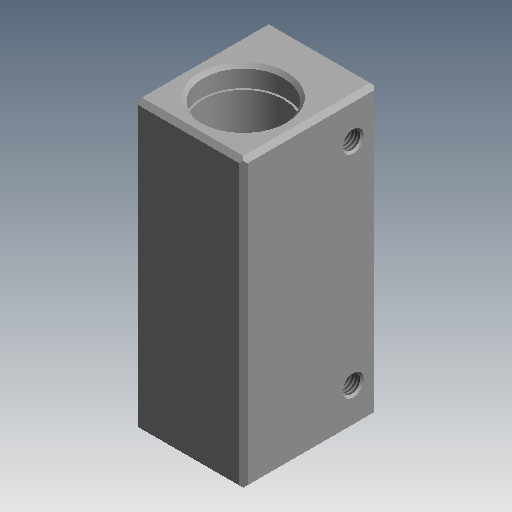
# Autodesk Inventor part: SLHSSW10_b
Saved by Autodesk Inventor 2020 (Build 240168000, 168)
## iProperties
Part Number: SLHSSW10_b
Material: 一般
Catalog Web Link: www.cadenas.de
Description: LHSSW, LHSSWF, SLHSSW, SLHSSWF_body-Linear Bushing Pillow Blocks - Standard Tall Blocks, Double
Vendor: MISUMI
Document SubType Name: Modeling
Designer: partserver
Manufacturer: MISUMI
Mass: 35.4256 g
Surface Area: 137.906 cm^2
Volume: 35.4256 cm^3
Density: 1 g/cm^3
Appearance: PSOLRGB-192-192-192
Category: PARTsolutions
Company: MISUMI
PSOL_IDENT_0: {$CADENAS_DATA\23d-libs\misumi\metric\04_linear_bushings\lhssw\lhssw_body.prj},196 {VTYP=3D},{NB=SLH
PSOL_IDENT_1: SSW10_b},{LINA=SLHSSW10},{NN=LHSSW, LHSSWF, SLHSSW, SLHSSWF_body},{DATE=30.11.2021 05:42:29},{GEOMDA
PSOL_IDENT_2: TE=06.10.2021 02:06:33},{VERSION=},{LINEID=90},{WBVAR=LB,GREASE},{WBNUMERIC=}  {NB=SLHSSW10_b},{LINA=
PSOL_IDENT_3: SLHSSW10},{KT=DUMMY},{PN=SLHSSW10},{TYPE=SLHSSW},{LB=SLMU},{LBALG= 'LMU', 'LMU', 'LMUF', 'LMUF', 'SL
PSOL_IDENT_4: MU', 'SLMU', 'SLMUS', 'SLMUS' },{GREASE=},{DDRR=10},{D=19},{RRTS=S},{RRNO=19},{S=4.0},{RRW=1.15},{RR
PSOL_IDENT_5: D=20.0},{RRC=0.8},{L=68},{L1=36},{L2=50},{HH=19},{W=26},{H=32},{LL=6},{M1=M6 (9.5)},{M13D=6},{M2=M5
PSOL_IDENT_6: (20)},{M23D=5},{C1=(1)},{C13D=1.0},{DD1TT=8x6 (for M4 Bolt)},{DD1=8.0},{TT=6.0}
NB: SLHSSW10_b
NN: LHSSW, LHSSWF, SLHSSW, SLHSSWF_body
NT: Linear Bushing Pillow Blocks - Standard Tall Blocks, Double
NBSYN: $PN._b
LINA: SLHSSW10
CATALOG: Misumi
PN: SLHSSW10
LB: SLMU
GREASE: Not Provided
DDRR: 10
D: 19
S: 4
L: 68
L1: 36
L2: 50
HH: 19
W: 26
H: 32
LL: 6
M1: M6 (9.5)
M2: M5 (20)
C1: (1)
C13D: 1
DD1TT: 8x6 (for M4 Bolt)
SUPPLIER: MISUMI
ARTICLENO: SLHSSW10_b
BOMINFO: SLHSSW10
CREATOR: CADENAS GmbH
Title: SLHSSW10
Author: Cadenas PARTsolutions
Comments: Linear Bushing Pillow Blocks - Standard Tall Blocks, Double
Autodesk Inventor part; units mm, degrees
sketch "Sketch_8" plane through (0, 0, 0) normal (1, 0, 0) x (0, 0, -1)
  line L0 (-34, 18) -> (-34, -12)
  line L1 (-34, -12) -> (-33, -13)
  line L2 (-33, -13) -> (33, -13)
  line L3 (33, -13) -> (34, -12)
  line L4 (34, -12) -> (34, 18)
  line L5 (34, 18) -> (33, 19)
  line L6 (33, 19) -> (-33, 19)
  line L7 (-33, 19) -> (-34, 18)
  constraints: 16 end point
extrude "Extrusion1" add sketch "Sketch_8" along normal mid plane 26
sketch "_____1" plane through (0, 0, 0) normal (0, 0, 1) x (1, 0, 0)
  line L0 (-14, -14) -> (14, -14)
  line L1 (14, -14) -> (14, 20)
  line L2 (14, 20) -> (-14, 20)
  line L3 (-14, 20) -> (-14, -14)
  line L4 (-13, 18) -> (-13, -12)
  line L5 (-13, -12) -> (-12, -13)
  line L6 (-12, -13) -> (12, -13)
  line L7 (12, -13) -> (13, -12)
  line L8 (13, -12) -> (13, 18)
  line L9 (13, 18) -> (12, 19)
  line L10 (12, 19) -> (-12, 19)
  line L11 (-12, 19) -> (-13, 18)
  constraints: 24 end point
extrude "Extrusion2" cut sketch "_____1" along normal mid plane 68
sketch "_____2" plane through (0, 0, 0) normal (0, 1, 0) x (1, 0, 0)
  line L0 (-14, -35) -> (14, -35)
  line L1 (14, -35) -> (14, 35)
  line L2 (14, 35) -> (-14, 35)
  line L3 (-14, 35) -> (-14, -35)
  line L4 (-13, 33) -> (-13, -33)
  line L5 (-13, -33) -> (-12, -34)
  line L6 (-12, -34) -> (12, -34)
  line L7 (12, -34) -> (13, -33)
  line L8 (13, -33) -> (13, 33)
  line L9 (13, 33) -> (12, 34)
  line L10 (12, 34) -> (-12, 34)
  line L11 (-12, 34) -> (-13, 33)
  constraints: 24 end point
extrude "Extrusion3" cut sketch "_____2" along normal mid plane 64
sketch "Sketch_1" plane through (0, 0, 0) normal (1, 0, 0) x (0, 0, -1)
  line L0 (34, 0) -> (-34, 0)
  line L1 (-34, 0) -> (-34, 10.3)
  line L2 (-34, 10.3) -> (-33.2, 9.5)
  line L3 (-33.2, 9.5) -> (-30, 9.5)
  line L4 (-30, 9.5) -> (-30, 10)
  line L5 (-30, 10) -> (-28.85, 10)
  line L6 (-28.85, 10) -> (-28.85, 9.5)
  line L7 (-28.85, 9.5) -> (28.85, 9.5)
  line L8 (28.85, 9.5) -> (28.85, 10)
  line L9 (28.85, 10) -> (30, 10)
  line L10 (30, 10) -> (30, 9.5)
  line L11 (30, 9.5) -> (33.2, 9.5)
  line L12 (33.2, 9.5) -> (34, 10.3)
  line L13 (34, 10.3) -> (34, 0)
  line L14 (34, 0) -> (-34, 0)
  constraints: 30 end point
revolve "Revolution1" cut sketch "Sketch_1" angle 360 about axis through (0, 0, -34) along (0, 0, -1)
sketch "Sketch5" plane through (-12, 19, -33) normal (0, 1, 0) x (1, 0, 0)
  point P0 (12, -15)
hole "Hole1" at (0, 19, -18) direction (0, -1, 0) diameter 4.917 depth 19 countersink diameter 6 countersink angle 90 thread size "M6x1" class "6H" standard "ISO Metric profile"
pattern_linear "Rectangular Pattern1" count 2 spacing 36 along (0, 0, 1) of "Hole1"
sketch "Sketch_3" plane through (0, 13, 0) normal (0, 1, 0) x (1, 0, 0)
  line L0 (13, 25) -> (-13, 25)
  line L1 (-13, 25) -> (-13, 27.5)
  line L2 (-13, 27.5) -> (-12.567, 27.067)
  line L3 (-12.567, 27.067) -> (6.567, 27.067)
  line L4 (6.567, 27.067) -> (7, 27.5)
  line L5 (7, 27.5) -> (7, 29)
  line L6 (7, 29) -> (13, 29)
  line L7 (13, 29) -> (13, 25)
  line L8 (13, 25) -> (-13, 25)
  constraints: 18 end point
revolve "Revolution2" cut sketch "Sketch_3" angle 360 about axis through (13, 13, -25) along (1, 0, 0)
thread "Thread1" size "M5x0.8" class "6H" standard "ISO Metric profile" full length
pattern_linear "Rectangular Pattern2" count 2 spacing 50 along (0, 0, 1) of "Revolution2"
ref_plane "to_bushings_XY" through (0, 0, 0) normal (0, 0, 1) x (1, 0, 0)
ref_plane "to_bushings_YZ" through (0, 0, 0) normal (1, 0, 0) x (0, 1, 0)
ref_plane "to_bushings_ZX" through (0, 0, 0) normal (0, 1, 0) x (0, 0, 1)
ref_plane "to_rring_l_XY" through (0, 0, 28.85) normal (0, 0, -1) x (1, 0, 0)
ref_plane "to_rring_l_YZ" through (0, 0, 28.85) normal (1, 0, 0) x (0, -1, 0)
ref_plane "to_rring_l_ZX" through (0, 0, 28.85) normal (0, -1, 0) x (0, 0, -1)
ref_plane "to_rring_r_XY" through (0, 0, -28.85) normal (0, 0, 1) x (-1, 0, 0)
ref_plane "to_rring_r_YZ" through (0, 0, -28.85) normal (-1, 0, 0) x (0, -1, 0)
ref_plane "to_rring_r_ZX" through (0, 0, -28.85) normal (0, -1, 0) x (0, 0, 1)
body "Solid1"
